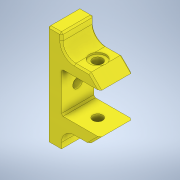
# Autodesk Inventor part: Part3
Saved by Autodesk Inventor 2021 (Build 250183000, 183)
## iProperties
Created: 2021-02-20
Part Number: Part3
Material: Generic
Document SubType Name: Modeling
Designer: dsdan
Density: 1 g/cm^3
Appearance: Default
Author: dsdan
Autodesk Inventor part; units mm, degrees
ref_plane "YZ Plane" through (0, 0, 0) normal (1, 0, 0) x (0, 1, 0)
ref_plane "XZ Plane" through (0, 0, 0) normal (0, 1, 0) x (-1, 0, 0)
ref_plane "XY Plane" through (0, 0, 0) normal (0, 0, 1) x (1, 0, 0)
sketch "Sketch1" plane through (0, 0, 0) normal (0, 0, 1) x (1, 0, 0)
  line L0 (-21.082, -58.8884) -> (-21.082, 26.0716) projected
  circle A0 centre (0, -16.4084) radius 3 projected
  arc A1 (-5.4102, -9.5755) -> (5.4102, -9.5755) centre (0, 0) ccw projected
  line L1 (-5.4102, -9.5755) -> (-5.4102, -5.6134) projected
  line L2 (-5.4102, -5.6134) -> (-3.7592, -5.6134) projected
  line L3 (-3.7592, -5.6134) -> (-3.2512, -5.1054) projected
  line L4 (-3.2512, -5.1054) -> (-3.2512, -3.9116) projected
  line L5 (-3.2512, -3.9116) -> (-11.4808, -3.9116) projected
  line L6 (-11.4808, -3.9116) -> (-12.4968, -4.9276) projected
  line L7 (-12.4968, -4.9276) -> (-12.4968, -13.1572) projected
  line L8 (-12.4968, -13.1572) -> (-11.303, -13.1572) projected
  line L9 (-11.303, -13.1572) -> (-10.795, -12.6492) projected
  line L10 (-10.795, -12.6492) -> (-10.795, -11.0109) projected
  line L11 (-10.795, -11.0109) -> (-6.8257, -11.0109) projected
  arc A2 (-6.8257, -21.8059) -> (-6.8257, -11.0109) centre (-16.4084, -16.4084) ccw projected
  line L12 (-6.8257, -21.8059) -> (-10.795, -21.8059) projected
  line L13 (-10.795, -21.8059) -> (-10.795, -20.1676) projected
  line L14 (-10.795, -20.1676) -> (-11.303, -19.6596) projected
  line L15 (-11.303, -19.6596) -> (-12.4968, -19.6596) projected
  line L16 (-12.4968, -19.6596) -> (-12.4968, -27.8892) projected
  line L17 (-12.4968, -27.8892) -> (-11.4808, -28.9052) projected
  line L18 (-11.4808, -28.9052) -> (-3.2512, -28.9052) projected
  line L19 (-3.2512, -28.9052) -> (-3.2512, -27.7114) projected
  line L20 (-3.2512, -27.7114) -> (-3.7592, -27.2034) projected
  line L21 (-3.7592, -27.2034) -> (-5.4102, -27.2034) projected
  line L22 (-5.4102, -27.2034) -> (-5.4102, -23.2413) projected
  arc A3 (5.4102, -23.2413) -> (-5.4102, -23.2413) centre (0, -32.8168) ccw projected
  line L23 (5.4102, -23.2413) -> (5.4102, -27.2034) projected
  line L24 (5.4102, -27.2034) -> (3.7592, -27.2034) projected
  line L25 (3.7592, -27.2034) -> (3.2512, -27.7114) projected
  line L26 (3.2512, -27.7114) -> (3.2512, -28.9052) projected
  line L27 (3.2512, -28.9052) -> (11.4808, -28.9052) projected
  line L28 (11.4808, -28.9052) -> (12.4968, -27.8892) projected
  line L29 (12.4968, -27.8892) -> (12.4968, -19.6596) projected
  line L30 (12.4968, -19.6596) -> (11.303, -19.6596) projected
  line L31 (11.303, -19.6596) -> (10.795, -20.1676) projected
  line L32 (10.795, -20.1676) -> (10.795, -21.8059) projected
  line L33 (10.795, -21.8059) -> (6.8257, -21.8059) projected
  arc A4 (6.8257, -11.0109) -> (6.8257, -21.8059) centre (16.4084, -16.4084) ccw projected
  line L34 (6.8257, -11.0109) -> (10.795, -11.0109) projected
  line L35 (10.795, -11.0109) -> (10.795, -12.6492) projected
  line L36 (10.795, -12.6492) -> (11.303, -13.1572) projected
  line L37 (11.303, -13.1572) -> (12.4968, -13.1572) projected
  line L38 (12.4968, -13.1572) -> (12.4968, -4.9276) projected
  line L39 (12.4968, -4.9276) -> (11.4808, -3.9116) projected
  line L40 (11.4808, -3.9116) -> (3.2512, -3.9116) projected
  line L41 (3.2512, -3.9116) -> (3.2512, -5.1054) projected
  line L42 (3.2512, -5.1054) -> (3.7592, -5.6134) projected
  line L43 (3.7592, -5.6134) -> (5.4102, -5.6134) projected
  line L44 (5.4102, -5.6134) -> (5.4102, -9.5755) projected
  circle A5 centre (-8.4963, -7.9121) radius 2.0193 projected
  circle A6 centre (8.4963, -24.9047) radius 2.0193 projected
  circle A7 centre (0, -16.4084) radius 3 projected
  circle A8 centre (-8.4963, -24.9047) radius 2.0193 projected
  circle A9 centre (8.4963, -7.9121) radius 2.0193 projected
  line L45 (-21.082, -47.8892) -> (-12.4968, -47.8892)
  line L46 (-12.4968, -47.8892) -> (-12.4968, -43.4052)
  line L47 (-12.4968, 10.5884) -> (-12.4968, 15.0724)
  line L48 (-12.4968, 15.0724) -> (-21.082, 15.0724)
  line L49 (-12.4968, -19.6596) -> (-12.4968, -13.1572)
  line L50 (-4.4968, -35.4052) -> (4.9808, -35.4052)
  line L51 (4.9808, -35.4052) -> (11.4808, -28.9052)
  line L52 (11.4808, -3.9116) -> (4.9808, 2.5884)
  line L53 (4.9808, 2.5884) -> (-4.4968, 2.5884)
  line L54 (3.2512, -28.9052) -> (-3.2512, -28.9052)
  line L55 (3.2512, -3.9116) -> (-3.2512, -3.9116)
  arc A10 (-4.4968, -35.4052) -> (-12.4968, -43.4052) centre (-4.4968, -43.4052) ccw
  arc A11 (-12.4968, 10.5884) -> (-4.4968, 2.5884) centre (-4.4968, 10.5884) ccw
  dimension "d0" = 20
  dimension "d1" = 20
  dimension "d2" = 45
  dimension "d3" = 6.5
  dimension "d4" = 6.5
  dimension "d5" = 45
  dimension "d6" = 8
  constraints: 22 end point, 5 point on line, 4 point on circle, 4 tangent, 3 perpendicular, 2 centre point, 2 collinear, 2 horizontal, 1 equal radius, 1 parallel
  measures "d0" distance of L6.end L47.end
  measures "d1" distance of L45.end L16.end
  measures "d2" angle of L27 L51
  measures "d3" distance between parallel lines of L27 L50
  measures "d4" horizontal distance of L39.end L52.end
  measures "d5" angle of L40 L52
  measures "d6" radius of A10
extrude "Extrusion1" add sketch "Sketch1" against normal blind 20 contours L0 L48 L47 A11 L53 L52 L40 L55 L5 L6 L7 L49 L16 L17 L18 L54 L27 L51 L50 A10 L46 L45
sketch "Sketch2" plane through (-4.4968, 2.5884, 0) normal (0, 1, 0) x (1, 0, 0)
  circle A0 centre (4.4968, 10) radius 5.1
  line L0 (0, 20) -> (9.4776, 20) projected
  line L1 (-6.984, 0) -> (15.9776, 0) projected
  point P0 (4.4968, 0)
  dimension "d9" = 10.2
  dimension "d17" = 10
  dimension "d18" = 10
  dimension "d19" = 11.4808
  dimension "d20" = 11.4808
  constraints: 1 centre point
  measures "d9" diameter of A0
  measures "d17" distance of point (4.497, 0) A0.centre
  measures "d18" distance from line of L0 A0.centre
  measures "d19" horizontal distance of L1.end A0.centre
  measures "d20" horizontal distance of L1.start A0.centre
extrude "Extrusion2" cut sketch "Sketch2" along normal blind 3 and the other way blind 1
sketch "Sketch3" plane through (0, 1.5884, -10) normal (0, 1, 0) x (1, 0, 0)
  circle A0 centre (0, 0) radius 3.05
  arc A1 (-4.4968, -2.406) -> (4.9808, -1.0962) centre (0, 0) ccw projected
  point P0 (0, -10)
  dimension "d14" = 6.1
  constraints: 1 centre point, 1 concentric
  measures "d14" diameter of A0
extrude "Extrusion3" cut sketch "Sketch3" against normal blind 10
sketch "Sketch4" plane through (-21.082, -47.8892, 0) normal (-1, 0, 0) x (0, 0, 1)
  line L0 (0, 62.9616) -> (0, 0) projected
  line L1 (0, 62.9616) -> (-20, 0) construction
  line L2 (0, 0) -> (-20, 0) projected
  line L3 (-20, 0) -> (-20, 62.9616) projected
  line L4 (0, 0) -> (-20, 62.9616) construction
  circle A0 centre (-10, 31.4808) radius 5.1
  point P0 (0, 47.8892)
  dimension "d21" = 10.2
  constraints: 4 end point, 1 centre point, 1 midpoint
  measures "d21" diameter of A0
extrude "Extrusion4" cut sketch "Sketch4" against normal blind 4.5
sketch "Sketch5" plane through (-16.582, -16.4084, -10) normal (-1, 0, 0) x (0, 0, 1)
  circle A0 centre (0, 0) radius 5.1 projected
  circle A1 centre (0, 0) radius 3.05
  point P0 (10, 16.4084)
  dimension "d24" = 6.1
  constraints: 1 centre point, 1 coincident
  measures "d24" diameter of A1
extrude "Extrusion5" cut sketch "Sketch5" against normal blind 10 contours A1
ref_plane "Work Plane1" through (-21.082, -16.4084, 0) normal (0, 1, 0) x (1, 0, 0)
mirror "Mirror1" about plane through (-21.082, -16.4084, 0) normal (0, 1, 0) of "Extrusion2", "Extrusion3"
chamfer "Chamfer1" distance 1 angle 45 23 edges at (-12.4968, 15.0724, -10) (-21.082, 15.0724, -10) (-12.4968, -47.8892, -10) (-21.082, -47.8892, -10) (-10.1537, 4.9315, 0) (-12.4968, 12.8304, 0) (0.242, 2.5884, 0) (-16.7894, 15.0724, 0) (-16.7894, 15.0724, -20) (-21.082, -16.4084, 0) (-21.082, -16.4084, -20) (-12.4968, 12.8304, -20) (-10.1537, 4.9315, -20) (0.242, 2.5884, -20) (0.242, -35.4052, -20) (-10.1537, -37.7483, -20) (-12.4968, -45.6472, -20) (-16.7894, -47.8892, -20) (-16.7894, -47.8892, 0) (8.2308, -0.6616, 0) (8.2308, -0.6616, -20) (8.2308, -32.1552, -20) (8.2308, -32.1552, 0)
equation "\"d17\" = d18"
equation "\"d19\" = d20"
body "Solid1"
